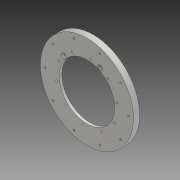
# Autodesk Inventor part: 1133_RU End Cap
Saved by Autodesk Inventor 2020 (Build 240168000, 168)
## iProperties
Created: 2019-03-26
Part Number: 1133_RU End Cap
Material: Generic
Document SubType Name: Modeling
Designer: e22ma
Density: 1 g/cm^3
Appearance: Default
Mass: 173.645 g
Surface Area: 523.308 cm^2
Volume: 173.645 cm^3
Author: e22ma
Autodesk Inventor part; units mm, degrees
ref_plane "Work Plane1" through (3.7155, 65.557, 54.6036) normal (0, -1, 0) x (0.9033475, 0, -0.4289095)
sketch "Sketch2" plane through (3.7155, 65.557, 54.6036) normal (0, -1, 0) x (0.9033475, 0, -0.4289095)
  circle A0 centre (-118.0349, 16.246) radius 4.7625 projected
  circle A1 centre (-57.404, 62.7698) radius 4.7625 projected
  circle A2 centre (-57.404, 0) radius 69.723 projected
  circle A3 centre (-57.404, 0) radius 57.404 projected
  circle A4 centre (-57.404, 0) radius 76.2 projected
  circle A5 centre (-57.404, 0) radius 84.2
  circle A6 centre (-107.7614, 37.4723) radius 1.0795 projected
  circle A7 centre (-50.1308, 62.3469) radius 1.0795 projected
  circle A8 centre (0.2267, 24.8747) radius 1.0795 projected
  circle A9 centre (-7.0466, -37.4723) radius 1.0795 projected
  circle A10 centre (-64.6772, -62.3469) radius 1.0795 projected
  circle A11 centre (-115.0347, -24.8747) radius 1.0795 projected
  circle A12 centre (-19.0569, -49.9749) radius 1.6475 projected
  circle A13 centre (-95.7511, 49.9749) radius 1.651 projected
  circle A14 centre (-120.1738, 0) radius 4.7625 projected
  circle A15 centre (-41.158, 60.6309) radius 4.7625 projected
  point P0 (20.0636, -50.9196)
  dimension "d0" = 8
  constraints: 1 centre point
  measures "d0" radial gap between concentric circles of A4 A5
extrude "Extrusion1" [suppressed]
ref_plane "Work Plane2" through (-48.1402, 113.182, 79.2247) normal (0, 0, 1) x (1, 0, 0)
sketch "Sketch4" plane through (-48.1402, 113.182, 79.2247) normal (0, 0, 1) x (1, 0, 0)
  line L0 (-76.2, -47.625) -> (76.2, -47.625) construction
  line L1 (0, -48.4188) -> (0, 19.2501)
  line L2 (-57.404, -47.625) -> (57.404, -47.625) construction
  line L3 (57.404, -47.625) -> (57.404, -48.4188)
  line L4 (57.404, -48.4188) -> (69.723, -48.4188)
  line L5 (69.723, -47.625) -> (-69.723, -47.625) construction
  line L6 (69.723, -48.4188) -> (69.723, -47.625)
  line L7 (69.723, -47.625) -> (76.2, -47.625)
  line L8 (76.2, -47.625) -> (76.2, -41.2188) construction
  line L9 (76.2, -41.2188) -> (96.2, -41.2188) construction
  line L10 (96.2, -41.2188) -> (96.2, -53.9188)
  line L11 (96.2, -53.9188) -> (57.404, -53.9188)
  line L12 (57.404, -53.9188) -> (57.404, -48.4188)
  line L13 (76.2, -44.6478) -> (80.1116, -44.6478)
  line L14 (80.1116, -44.6478) -> (80.1116, -41.2188)
  line L15 (80.1116, -41.2188) -> (76.2, -41.2188) construction
  line L16 (76.2, -41.2188) -> (76.2, -44.6478) construction
  line L17 (76.2, -44.6478) -> (76.2, -47.625)
  line L18 (76.2, -41.2188) -> (76.2, -41.2188) construction
  line L19 (96.2, -41.2188) -> (80.1116, -41.2188)
  point P0 (48.1402, -113.182)
  dimension "d4" = 20
  dimension "d9" = 3.9116
  dimension "d10" = 3.429
  dimension "d14" = 12.7
  dimension "d15" = 5.5
  dimension "d32" = 0.7937
  constraints: 34 end point, 7 perpendicular, 3 point on line, 3 vertical, 2 horizontal, 2 parallel, 1 collinear
  measures "d4" distance of L8.end L9.end
  measures "d9" distance of L15.end L14.end
  measures "d10" distance of L14.end L13.end
  measures "d14" distance between parallel lines of L9 L11
  measures "d15" distance between parallel lines of L4 L11
  measures "d32" distance between parallel lines of L7 L4
revolve "Revolution1" add sketch "Sketch4" angle 360 about axis through (-48.1402, 64.7633, 79.2247) along (0, 1, 0) separate body
sketch "Sketch5" plane through (-48.1402, 59.2633, 79.2247) normal (0, -1, 0) x (1, 0, 0)
  circle A0 centre (0, 0) radius 57.404 projected
  circle A1 centre (26.9225, 56.7029) radius 4.7625 projected
  circle A2 centre (40.681, 47.8027) radius 4.7625 projected
  circle A3 centre (-56.7029, 26.9225) radius 4.7625 projected
  circle A4 centre (-47.8027, 40.681) radius 4.7625 projected
  circle A5 centre (0, 0) radius 69.723 projected
  point P0 (48.1402, -79.2247)
extrude "Extrusion2" cut sketch "Sketch5" against normal through all contours A1 | A4
ref_plane "Work Plane3" through (-48.1402, 113.182, 79.2247) normal (0, 0, 1) x (1, 0, 0)
sketch "Sketch8" plane through (-48.1402, 71.9633, 79.2247) normal (0, 1, 0) x (1, 0, 0)
  circle A0 centre (0, 0) radius 96.2 projected
  line L0 (96.2, 0) -> (76.2, 0)
  circle A1 centre (0, 0) radius 76.2
  point P0 (48.1402, 79.2247)
  point P1 (86.2, 0)
  dimension "d39" = 152.4
  constraints: 3 horizontal alignment, 2 end point, 1 coincident, 1 horizontal, 1 midpoint, 3 other
hole "Hole1" at (38.0598, 71.9633, 79.2247) direction (0, -1, 0) diameter 3.683 end through all thread size "10-24 UNC" class "2B" standard "ANSI Unified Screw Threads"
pattern_circular "Circular Pattern1" count 10 over 360 about axis through (-48.1402, 65.6133, 79.2247) along (0, -1, 0) of "Hole1"
sketch "Sketch12" plane through (-48.1402, 64.7633, 79.2247) normal (0, -1, 0) x (1, 0, 0)
  circle A0 centre (-62.4688, -11.7461) radius 1.8415 projected
  circle A1 centre (-30.4751, 55.7816) radius 1.8415 projected
  circle A2 centre (62.4688, 11.7461) radius 1.8415 projected
  circle A3 centre (30.4751, -55.7816) radius 1.8415 projected
  circle A4 centre (8.1327, 63.0411) radius 1.8415 projected
  circle A5 centre (-8.1327, -63.0411) radius 1.8415 projected
  circle A6 centre (57.4425, -27.2155) radius 1.8415 projected
  circle A7 centre (43.6341, 46.221) radius 1.8415 projected
  circle A8 centre (-57.4425, 27.2155) radius 1.8415 projected
  circle A9 centre (-43.6341, -46.221) radius 1.8415 projected
  circle A10 centre (0, 0) radius 57.404 projected
  circle A11 centre (0, 0) radius 72.898 projected
  circle A12 centre (26.9225, 56.7029) radius 4.7625 projected
  circle A13 centre (-47.8027, 40.681) radius 4.7625 projected
  circle A14 centre (0, 0) radius 57.404 projected
  circle A15 centre (0, 0) radius 69.723 projected
  point P0 (48.1402, -79.2247)
extrude "Extrusion6" cut sketch "Sketch12" along normal through all contours A0 | A1 | A2 | A3 | A4 | A5 | A6 | A7 | A8 | A9
sketch "Sketch13" plane through (-48.1402, 71.9633, 79.2247) normal (0, 1, 0) x (1, 0, 0)
  circle A0 centre (0, 0) radius 96.2 projected
  circle A1 centre (0, 0) radius 76.454
  point P0 (48.1402, 79.2247)
  dimension "d35" = 152.908
  constraints: 1 centre point, 1 coincident
  measures "d35" diameter of A1
extrude "Extrusion7" cut sketch "Sketch13" against normal up to surface (6.4063 mm away) contours A1
body "Solid1"
body "Solid2"
